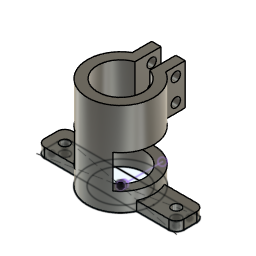
motor clamp v3 (Autodesk Fusion 360 design; units mm, degrees)
Autodesk Fusion 360 part; units mm, degrees
note: some values were not read from the file. Set by a fixed rule: which sketch regions a step uses.
sketch "Sketch1" plane through (0, 0, 0) normal (0, 0, 1) x (1, 0, 0)
  line L0 (33.5, -7.5) -> (-33.5, -7.5)
  line L1 (-37.5, -3.5) -> (-37.5, 3.5)
  line L2 (-33.5, 7.5) -> (33.5, 7.5)
  line L3 (37.5, 3.5) -> (37.5, -3.5)
  line L4 (37.5, -7.5) -> (-37.5, 7.5) construction
  line L5 (-37.5, -7.5) -> (37.5, 7.5) construction
  circle A0 centre (0, 0) radius 12.75
  circle A1 centre (0, 0) radius 17.75
  circle A2 centre (30, 0) radius 2.5
  circle A3 centre (-30, 0) radius 2.5
  line L6 (0, 1.75) -> (0, 22.5)
  arc A4 (37.5, 3.5) -> (33.5, 7.5) centre (33.5, 3.5) ccw
  arc A5 (33.5, -7.5) -> (37.5, -3.5) centre (33.5, -3.5) ccw
  arc A6 (-37.5, -3.5) -> (-33.5, -7.5) centre (-33.5, -3.5) ccw
  arc A7 (-33.5, 7.5) -> (-37.5, 3.5) centre (-33.5, 3.5) ccw
  dimension "d1" = 75
  dimension "d2" = 15
  dimension "d3" = 25.5
  dimension "d4" = 35.5
  dimension "d5" = 5
  dimension "d6" = 5
  dimension "d7" = 60
  dimension "d8" = 7.5
  dimension "d13" = 4
  dimension "d14" = 4
  constraint horizontal L0
  constraint perpendicular L0 L1
  constraint parallel L0 L2
  constraint parallel L1 L3
  constraint coincident L4 A0.centre
  constraint coincident L5 A0.centre
  constraint coincident A0.centre A1.centre
  constraint concentric A0 A1
  constraint symmetric A2.centre A3.centre L6
  constraint coincident L5.end L2
  constraint coincident L5.end L3
  constraint tangent L2 A4
  constraint tangent L3 A4
  constraint coincident L4.start L3
  constraint coincident L4.start L0
  constraint tangent L3 A5
  constraint tangent L0 A5
  constraint coincident L5.start L0
  constraint coincident L5.start L1
  constraint tangent L0 A6
  constraint tangent L1 A6
  constraint equal A5 A6
  constraint coincident L4.end L2
  constraint coincident L4.end L1
  constraint tangent L2 A7
  constraint tangent L1 A7
  constraint equal A5 A7
  measures "d1" distance of L4.end L5.end
  measures "d2" distance of L5.start L4.end
  measures "d3" diameter of A0
  measures "d4" diameter of A1
  measures "d5" diameter of A2
  measures "d6" diameter of A3
  measures "d7" distance of A2.centre A3.centre
  measures "d8" distance of L2 A2.centre
  measures "d13" radius of A4
  measures "d14" radius of A5
extrude "Extrude1" add sketch "Sketch1" along normal blind 5 contours L0 L2 L3 A1 A4 A5 | L0 L2 A0 A1 | L0 L2 A0 A1 | L0 L1 L2 A1 A6 A7 makes body 1 at (-24.5017, 5.2186, 0) makes body 2 at (24.5017, -5.2186, 5)
extrude "Extrude2" add sketch "Sketch1" along normal blind 10 contours L0 A0 A1 | L0 L2 A0 A1 | L0 L2 A0 A1 | L2 A0 A1 L6 | L2 A0 A1 L6 bodies 1 2
sketch "Sketch2" plane through (0, 0, 10) normal (0, 0, 1) x (-1, 0, 0)
  circle A0 centre (0, 0) radius 12.75
  circle A1 centre (0, 0) radius 17.75
  line L0 (-3.5817, 12.2366) -> (-10.317, 14.4438)
  circle A2 centre (0, 0) radius 12.75
  circle A3 centre (0, 0) radius 17.75
  line L1 (0, -1.75) -> (0, -22.5)
  line L2 (3.5817, 12.2366) -> (10.317, 14.4438)
  dimension "d17" = 7.0877
  constraint coincident A0 L0.start
  constraint coincident A1 L0.end
  constraint coincident A0.centre A1.centre
  constraint concentric A2 A3
  constraint coincident L0.end A3
  constraint symmetric L0.start L1 L2.start
  constraint symmetric L0.end L1 L2.end
  measures "d17" distance of L0.start L0.end
extrude "Extrude3" add sketch "Sketch2" along normal blind 18 contours A0 A1 L0 A2 A3 L2 bodies 1
sketch "Sketch3" plane through (0, 0, 28) normal (0, 0, 1) x (-1, 0, 0)
  arc A0 (3.5817, 12.2366) -> (-3.5817, 12.2366) centre (0, 0) ccw
  line L0 (3.5817, 12.2366) -> (10.317, 14.4438)
  arc A1 (10.317, 14.4438) -> (-10.317, 14.4438) centre (0, 0) ccw
  line L1 (-10.317, 14.4438) -> (-3.5817, 12.2366)
  circle A2 centre (0, 0) radius 12.4
  circle A3 centre (0, 0) radius 17.75
  line L2 (4, -11.7371) -> (9, -11.7371)
  line L3 (9, -11.7371) -> (9, -25.7371)
  line L4 (9, -25.7371) -> (4, -25.7371)
  line L5 (4, -25.7371) -> (4, -11.7371)
  line L6 (0, -1.75) -> (0, -22.5)
  line L7 (-4, -25.7371) -> (-4, -11.7371)
  line L8 (-9, -11.7371) -> (-9, -25.7371)
  line L9 (-9, -25.7371) -> (-4, -25.7371)
  line L10 (-4, -11.7371) -> (-9, -11.7371)
  dimension "d18" = 24.8
  dimension "d19" = 35.5
  dimension "d22" = 5
  dimension "d23" = 14
  dimension "d24" = 18
  constraint concentric A0 A2
  constraint concentric A2 A3
  constraint horizontal L2
  constraint vertical L3
  constraint horizontal L4
  constraint vertical L5
  constraint coincident A2 L2.start
  constraint symmetric L2.start L6 L7.end
  constraint symmetric L2.end L6 L8.start
  constraint symmetric L3.end L6 L8.end
  constraint symmetric L4.end L6 L7.start
  measures "d18" diameter of A2
  measures "d19" diameter of A3
  measures "d22" distance of L2.start L2.end
  measures "d23" distance of L2.end L3.end
  measures "d24" distance of L3 L8
extrude "Extrude4" add sketch "Sketch3" along normal blind 22 contours A0 L0 L1 A2 A3 L2 L3 L8 L10 | A0 L0 A1 L1 A3 | A3 L7 L8 L10 | A3 L7 L8 L9 | A3 L3 L4 L5 | A3 L2 L3 L5 bodies 1
hole "Hole1" at (-9, 20.7371, 45) direction (1, 0, 0) diameter 5 depth 23 tip angle 180 bodies 1
hole "Hole2" at (-9, 20.7371, 33) direction (1, 0, 0) diameter 5 depth 23 tip angle 180 bodies 1
equation "d4 = d3 + 10 mm"
equation "d8 = d2 / 2"
